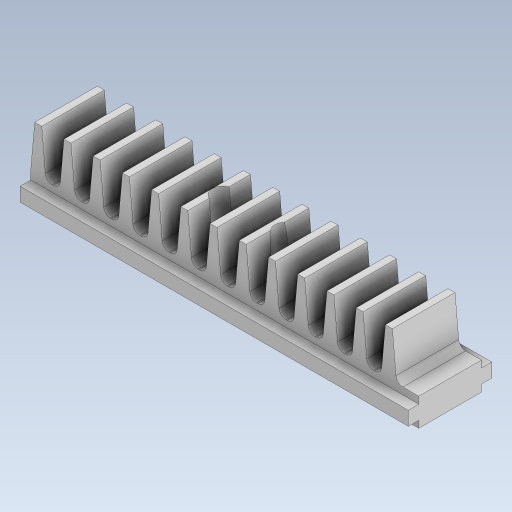
# Autodesk Inventor part: Rack Lifter
Saved by Autodesk Inventor 2023.5 (Build 275446000, 446)
## iProperties
Created: 2025-09-02
Part Number: Rack Lifter
Material: Generic
Document SubType Name: Modeling
Designer: Guntur
Density: 1 g/cm^3
Appearance: Default
Author: Guntur
## iProperties of the stored document Rack Lifter_3DPrint.ipt
Created: 2025-09-02
Part Number: Rack Lifter_3DPrint
Material: Generic
Document SubType Name: Modeling
Designer: Guntur
Density: 1 g/cm^3
Appearance: Default
Author: Guntur
Autodesk Inventor part; units mm, degrees
ref_plane "YZ Plane" through (0, 0, 0) normal (1, 0, 0) x (0, 1, 0)
ref_plane "XZ Plane" through (0, 0, 0) normal (0, 1, 0) x (-1, 0, 0)
sketch "Sketch1" plane through (0, 0, 0) normal (0, 0, 1) x (1, 0, 0)
  line L0 (0, 14.654) -> (0, -13.4329) construction
  line L1 (-3, 0.0203) -> (54.693, 0.0203)
  line L2 (-3, 3.5203) -> (54.693, 3.5203)
  line L3 (-3, 6.5203) -> (54.693, 6.5203)
  arc A0 (-0.5, 6.5203) -> (-1.1, 0.0203) centre (654.7575, -57.2427) ccw
  arc A1 (1.1, 0.0203) -> (0.5, 6.5203) centre (-654.7575, -57.2427) ccw
  line L4 (-1.1, 0.0203) -> (54.693, 0.0203)
  line L5 (54.693, 0.0203) -> (54.693, -3.9797)
  line L6 (54.693, -3.9797) -> (-1.1, -3.9797)
  line L7 (-1.1, -3.9797) -> (-1.1, 0.0203)
  point P0 (0, 0)
  point P1 (-0.785, 3.5203)
  point P2 (0.785, 3.5203)
  point P3 (1.1, 0.0203)
  point P4 (0.5, 6.5203)
  dimension "d29" = 3.5
  dimension "d30" = 3
  dimension "d31" = 3
  dimension "d32" = 1.57
  dimension "d33" = 0.785
  dimension "d34" = 1
  dimension "d35" = 2.2
  dimension "d36" = 4
  constraints: 16 end point, 5 point on circle, 4 horizontal, 4 point on line, 3 symmetric about line, 2 centre point, 2 parallel, 1 horizontal alignment, 1 perpendicular, 1 vertical, 1 other
  measures "d29" distance between parallel lines of L2 L1
  measures "d30" distance between parallel lines of L2 L3
  measures "d31" distance from line of L0 L1.start
  measures "d32" distance of point (0.785, 3.52) point (-0.785, 3.52)
  measures "d33" distance from line of L0 point (-0.785, 3.52)
  measures "d34" distance of A1.end A0.start
  measures "d35" distance of A1.start L4.start
  measures "d36" distance of L4.end L5.end
extrude "Extrusion1" add sketch "Sketch1" along normal blind 9 contours L1 L5 L6 L7
extrude "Extrusion2" add sketch "Sketch1" along normal blind 9 contours A0 L2 A1 L1 | A0 L3 A1 L2
fillet "Fillet1" radius 1 2 edges at (1.1, 0.0203, 4.5) (-1.1, 0.0203, 4.5)
pattern_linear "Rectangular Pattern1" count 13 spacing 4.2 along (1, 0, 0) of "Extrusion2", "Fillet1"
fillet_without_effect "Fillet2"
ref_plane "Work Plane1" through (36.7802, 0.932, 4.5) normal (0, 0, 1) x (1, 0, 0)
sketch "Sketch2" plane through (36.7802, 0.932, 4.5) normal (0, 0, 1) x (1, 0, 0)
  line L0 (-37.8802, -0.9552) -> (-37.8802, -4.9116) projected
  line L1 (17.9128, -4.9116) -> (17.9128, -0.9116) projected
  line L2 (-37.8802, -1.9116) -> (17.9128, -1.9116)
  line L3 (17.9128, -1.9116) -> (17.9128, -3.9116)
  line L4 (17.9128, -3.9116) -> (-37.8802, -3.9116)
  line L5 (-37.8802, -3.9116) -> (-37.8802, -1.9116)
  point P0 (-36.7802, -0.932)
  point P1 (-37.8802, -3.9116)
  dimension "d46" = 2
  dimension "d47" = 1
  constraints: 8 end point, 2 parallel, 2 point on line, 1 horizontal, 1 perpendicular
  measures "d46" distance of L2.end L3.end
  measures "d47" distance of L0.end L4.end
extrude "Extrusion3" add sketch "Sketch2" along normal mid plane 12
sketch "Sketch3" plane through (-1.1, -3.9797, 0) normal (0, -1, 0) x (1, 0, 0)
  line L0 (23.1198, 0) -> (23.1198, 9) projected
  circle A0 centre (23.1198, 4.5) radius 1.5
  circle A1 centre (32.1198, 4.5) radius 1.5
  point P0 (1.1, 0)
  dimension "d50" = 3
  dimension "d51" = 3
  dimension "d52" = 9
  constraints: 2 centre point, 1 midpoint
  measures "d50" diameter of A0
  measures "d51" diameter of A1
  measures "d52" distance of A1.centre A0.centre
extrude "Extrusion4" cut sketch "Sketch3" against normal blind 12
body "Solid1"
